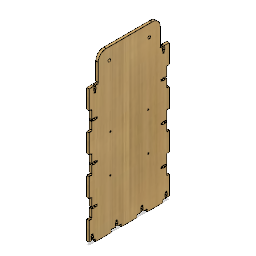
Square-plate-IIIS-electronics-rev1_8mm v1 (Autodesk Fusion 360 design; units mm, degrees)
Autodesk Fusion 360 part; units mm, degrees
sketch "Basic shape" plane through (0, 0, 0) normal (1, 0, 0) x (0, 0, -1)
  line L0 (-117.75, 0) -> (117.75, 0)
  line L1 (117.75, 0) -> (117.75, 417)
  line L2 (117.75, 417) -> (-117.75, 417)
  line L3 (-117.75, 417) -> (-117.75, 0)
  line L4 (-97.5, 417) -> (97.5, 417)
  line L5 (97.5, 417) -> (97.5, 500)
  line L6 (97.5, 500) -> (-97.5, 500)
  line L7 (-97.5, 500) -> (-97.5, 417)
  line L8 (117.75, 0) -> (125.75, 0)
  line L9 (125.75, 0) -> (125.75, 60)
  line L10 (125.75, 60) -> (117.75, 60)
  line L11 (117.75, 60) -> (117.75, 0)
  line L12 (117.75, 119) -> (125.75, 119)
  line L13 (125.75, 119) -> (125.75, 179)
  line L14 (125.75, 179) -> (117.75, 179)
  line L15 (117.75, 179) -> (117.75, 119)
  line L16 (117.75, 238) -> (125.75, 238)
  line L17 (125.75, 238) -> (125.75, 298)
  line L18 (125.75, 298) -> (117.75, 298)
  line L19 (117.75, 298) -> (117.75, 238)
  line L20 (117.75, 357) -> (125.75, 357)
  line L21 (125.75, 357) -> (125.75, 417)
  line L22 (125.75, 417) -> (117.75, 417)
  line L23 (117.75, 417) -> (117.75, 357)
  line L24 (-117.75, 0) -> (-55.75, 0)
  line L25 (-55.75, 0) -> (-55.75, -8)
  line L26 (-55.75, -8) -> (-105.75, -8)
  line L27 (-25, 0) -> (25, 0)
  line L28 (25, 0) -> (25, -8)
  line L29 (25, -8) -> (-25, -8)
  line L30 (-25, -8) -> (-25, 0)
  line L31 (117.75, 0) -> (55.75, 0)
  line L32 (55.75, 0) -> (55.75, -8)
  line L33 (55.75, -8) -> (105.75, -8)
  line L34 (-55.75, -8) -> (-25, -8) construction
  line L35 (25, -8) -> (55.75, -8) construction
  line L36 (-117.75, 0) -> (-125.75, 0)
  line L37 (-125.75, 0) -> (-125.75, 60)
  line L38 (-125.75, 60) -> (-117.75, 60)
  line L39 (-117.75, 60) -> (-117.75, 0)
  line L40 (-117.75, 119) -> (-125.75, 119)
  line L41 (-125.75, 119) -> (-125.75, 179)
  line L42 (-125.75, 179) -> (-117.75, 179)
  line L43 (-117.75, 179) -> (-117.75, 119)
  line L44 (-117.75, 238) -> (-125.75, 238)
  line L45 (-125.75, 238) -> (-125.75, 298)
  line L46 (-125.75, 298) -> (-117.75, 298)
  line L47 (-117.75, 298) -> (-117.75, 238)
  line L48 (-117.75, 357) -> (-125.75, 357)
  line L49 (-125.75, 357) -> (-125.75, 417)
  line L50 (-125.75, 417) -> (-117.75, 417)
  line L51 (-117.75, 417) -> (-117.75, 357)
  line L52 (125.75, 60) -> (125.75, 119) construction
  line L53 (125.75, 179) -> (125.75, 238) construction
  line L54 (-125.75, 60) -> (-125.75, 119) construction
  line L55 (-125.75, 179) -> (-125.75, 238) construction
  line L56 (-105.75, 0) -> (-105.75, -8)
  line L57 (105.75, -8) -> (105.75, 0)
  line L58 (97.5, 417) -> (125.75, 417)
  line L59 (-125.75, 417) -> (-97.5, 417)
  line L60 (-125.75, 357) -> (-125.75, 298) construction
  line L61 (125.75, 357) -> (125.75, 298) construction
  dimension "d1" = 235.5
  dimension "d2" = 417
  dimension "d3" = 83
  dimension "d4" = 195
  dimension "d9" = 60
  dimension "d10" = 60
  dimension "d11" = 60
  dimension "d12" = 60
  dimension "d16" = 50
  dimension "d20" = 8
  dimension "d21" = 8
  dimension "d22" = 60
  dimension "d24" = 60
  dimension "d26" = 60
  dimension "d28" = 60
  dimension "d29" = 8
  dimension "d30" = 8
  dimension "d81" = 8
  dimension "d82" = 20
  dimension "d83" = 20
  dimension "d357" = 50
  dimension "d358" = 50
  dimension "d359" = 30.75
  dimension "d360" = 30.75
  measures "d2" distance of origin
  measures "d22" distance of origin
  measures "d81" distance of L0 L26
  measures "d83" distance of origin
extrude "Extrude1" add sketch "Basic shape" along normal blind 8
sketch "T slots horizontal" plane through (8, 0, 0) normal (1, 0, 0) x (0, 0, -1)
  line L0 (-117.75, 357) -> (-117.75, 298)
  line L1 (-117.75, 298) -> (-125.75, 298)
  line L2 (-125.75, 298) -> (-125.75, 238)
  line L3 (-125.75, 238) -> (-117.75, 238)
  line L4 (-117.75, 238) -> (-117.75, 179)
  line L5 (-117.75, 179) -> (-125.75, 179)
  line L6 (-125.75, 179) -> (-125.75, 119)
  line L7 (-125.75, 119) -> (-117.75, 119)
  line L8 (-117.75, 119) -> (-117.75, 60)
  line L9 (-117.75, 60) -> (-125.75, 60)
  line L10 (-125.75, 60) -> (-125.75, 0)
  line L11 (-125.75, 0) -> (-117.75, 0)
  line L12 (-105.75, -8) -> (-55.75, -8)
  line L13 (-55.75, -8) -> (-55.75, 0)
  line L14 (-117.75, 0) -> (-105.75, 0)
  line L15 (-25, 0) -> (-25, -8)
  line L16 (-25, -8) -> (25, -8)
  line L17 (25, -8) -> (25, 0)
  line L18 (25, 0) -> (55.75, 0)
  line L19 (55.75, 0) -> (55.75, -8)
  line L20 (55.75, -8) -> (105.75, -8)
  line L21 (105.75, 0) -> (125.75, 0)
  line L22 (125.75, 0) -> (125.75, 60)
  line L23 (125.75, 60) -> (117.75, 60)
  line L24 (117.75, 60) -> (117.75, 119)
  line L25 (117.75, 119) -> (125.75, 119)
  line L26 (125.75, 119) -> (125.75, 179)
  line L27 (125.75, 179) -> (117.75, 179)
  line L28 (117.75, 179) -> (117.75, 238)
  line L29 (117.75, 238) -> (125.75, 238)
  line L30 (125.75, 238) -> (125.75, 298)
  line L31 (125.75, 298) -> (117.75, 298)
  line L32 (117.75, 298) -> (117.75, 357)
  line L33 (117.75, 357) -> (125.75, 357)
  line L34 (125.75, 357) -> (125.75, 417)
  line L35 (125.75, 417) -> (97.5, 417)
  line L36 (97.5, 417) -> (97.5, 500)
  line L37 (97.5, 500) -> (-97.5, 500)
  line L38 (-97.5, 500) -> (-97.5, 417)
  line L39 (-97.5, 417) -> (-125.75, 417)
  line L40 (-125.75, 417) -> (-125.75, 357)
  line L41 (-125.75, 357) -> (-117.75, 357)
  line L42 (-41.885, 0) -> (-37.865, 0)
  line L43 (-37.865, 0) -> (-37.865, 17.5)
  line L44 (-37.865, 17.5) -> (-41.885, 17.5)
  line L45 (-41.885, 17.5) -> (-41.885, 0)
  line L46 (-43.355, 12.5) -> (-36.355, 12.5)
  line L47 (-36.355, 12.5) -> (-36.355, 5)
  line L48 (-36.355, 5) -> (-43.355, 5)
  line L49 (-43.355, 5) -> (-43.355, 12.5)
  line L50 (-109.635, 417) -> (-105.615, 417)
  line L51 (-105.615, 417) -> (-105.615, 397)
  line L52 (-105.615, 397) -> (-109.635, 397)
  line L53 (-109.635, 397) -> (-109.635, 417)
  line L54 (-111.105, 412) -> (-104.105, 412)
  line L55 (-104.105, 412) -> (-104.105, 404.5)
  line L56 (-104.105, 404.5) -> (-111.105, 404.5)
  line L57 (-111.105, 404.5) -> (-111.105, 412)
  line L58 (-113.74, 0) -> (-113.74, 17.5)
  line L59 (-117.76, 17.5) -> (-117.76, 0)
  line L60 (-113.74, 17.5) -> (-117.76, 17.5)
  line L61 (-119.23, 5) -> (-119.23, 12.5)
  line L62 (-112.23, 5) -> (-119.23, 5)
  line L63 (-117.76, 0) -> (-113.74, 0)
  line L64 (-112.23, 12.5) -> (-112.23, 5)
  line L65 (-119.23, 12.5) -> (-112.23, 12.5)
  line L66 (-105.75, 0) -> (-105.75, -8)
  line L67 (105.75, -8) -> (105.75, 0)
  line L68 (-55.75, 0) -> (-25, 0)
  dimension "d31" = 4.02
  dimension "d32" = 7
  dimension "d33" = 1.51
  dimension "d34" = 5
  dimension "d35" = 17.5
  dimension "d36" = 7.5
  dimension "d37" = 4.02
  dimension "d38" = 20
  dimension "d39" = 7.5
  dimension "d40" = 1.51
  dimension "d41" = 7
  dimension "d42" = 5
  dimension "d66" = 4.02
  dimension "d67" = 7
  dimension "d68" = 1.51
  dimension "d69" = 5
  dimension "d70" = 17.5
  dimension "d71" = 7.5
  dimension "d80" = 10.125
  dimension "d86" = 14.625
  dimension "d90" = 10
  measures "d33" distance of L43
  measures "d34" distance of origin
  measures "d35" distance of origin
  measures "d68" distance of L58
  measures "d69" distance of origin
  measures "d70" distance of origin
  measures "d90" distance of origin L66
extrude "Extrude2" cut sketch "T slots horizontal" against normal through all contours L39 L50 L51 L53 L54 | L51 L53 L54 L56 | L53 L54 L56 L57 | L51 L54 L55 L56 | L51 L52 L53 L56 | L11 L14 L58 L59 L62 L63 | L59 L61 L62 L65 | L58 L59 L62 L65 | L58 L59 L60 L65 | L58 L62 L64 L65 | L42 L43 L45 L48 L68 | L45 L46 L48 L49 | L43 L45 L46 L48 | L43 L46 L47 L48 | L43 L44 L45 L46
mirror "Mirror1" about plane through (0, 0, 0) normal (0, 0, 1) of "Extrude2"
sketch "T slots vertical" plane through (8, 0, 0) normal (1, 0, 0) x (0, 0, -1)
  line L0 (37.865, 0) -> (37.865, 5)
  line L1 (37.865, 5) -> (36.355, 5)
  line L2 (36.355, 5) -> (36.355, 12.5)
  line L3 (36.355, 12.5) -> (37.865, 12.5)
  line L4 (37.865, 12.5) -> (37.865, 17.5)
  line L5 (37.865, 17.5) -> (41.885, 17.5)
  line L6 (41.885, 17.5) -> (41.885, 12.5)
  line L7 (41.885, 12.5) -> (43.355, 12.5)
  line L8 (43.355, 12.5) -> (43.355, 5)
  line L9 (43.355, 5) -> (41.885, 5)
  line L10 (41.885, 5) -> (41.885, 0)
  line L11 (41.885, 0) -> (55.75, 0)
  line L12 (55.75, 0) -> (55.75, -8)
  line L13 (55.75, -8) -> (105.75, -8)
  line L14 (105.75, 0) -> (113.74, 0)
  line L15 (125.75, 0) -> (125.75, 60)
  line L16 (125.75, 60) -> (117.75, 60)
  line L17 (117.75, 60) -> (117.75, 119)
  line L18 (117.75, 119) -> (125.75, 119)
  line L19 (125.75, 119) -> (125.75, 179)
  line L20 (125.75, 179) -> (117.75, 179)
  line L21 (117.75, 179) -> (117.75, 238)
  line L22 (117.75, 238) -> (125.75, 238)
  line L23 (125.75, 238) -> (125.75, 298)
  line L24 (125.75, 298) -> (117.75, 298)
  line L25 (117.75, 298) -> (117.75, 357)
  line L26 (117.75, 357) -> (125.75, 357)
  line L27 (125.75, 357) -> (125.75, 417)
  line L28 (125.75, 417) -> (109.635, 417)
  line L29 (109.635, 417) -> (109.635, 412)
  line L30 (109.635, 412) -> (111.105, 412)
  line L31 (111.105, 412) -> (111.105, 404.5)
  line L32 (111.105, 404.5) -> (109.635, 404.5)
  line L33 (109.635, 404.5) -> (109.635, 397)
  line L34 (109.635, 397) -> (105.615, 397)
  line L35 (105.615, 397) -> (105.615, 404.5)
  line L36 (105.615, 404.5) -> (104.105, 404.5)
  line L37 (104.105, 404.5) -> (104.105, 412)
  line L38 (104.105, 412) -> (105.615, 412)
  line L39 (105.615, 412) -> (105.615, 417)
  line L40 (105.615, 417) -> (97.5, 417)
  line L41 (97.5, 417) -> (97.5, 500)
  line L42 (97.5, 500) -> (-97.5, 500)
  line L43 (-97.5, 500) -> (-97.5, 417)
  line L44 (-97.5, 417) -> (-105.615, 417)
  line L45 (-105.615, 417) -> (-105.615, 412)
  line L46 (-105.615, 412) -> (-104.105, 412)
  line L47 (-104.105, 412) -> (-104.105, 404.5)
  line L48 (-104.105, 404.5) -> (-105.615, 404.5)
  line L49 (-105.615, 404.5) -> (-105.615, 397)
  line L50 (-105.615, 397) -> (-109.635, 397)
  line L51 (-109.635, 397) -> (-109.635, 404.5)
  line L52 (-109.635, 404.5) -> (-111.105, 404.5)
  line L53 (-111.105, 404.5) -> (-111.105, 412)
  line L54 (-111.105, 412) -> (-109.635, 412)
  line L55 (-109.635, 412) -> (-109.635, 417)
  line L56 (-109.635, 417) -> (-125.75, 417)
  line L57 (-125.75, 417) -> (-125.75, 357)
  line L58 (-125.75, 357) -> (-117.75, 357)
  line L59 (-117.75, 357) -> (-117.75, 298)
  line L60 (-117.75, 298) -> (-125.75, 298)
  line L61 (-125.75, 298) -> (-125.75, 238)
  line L62 (-125.75, 238) -> (-117.75, 238)
  line L63 (-117.75, 238) -> (-117.75, 179)
  line L64 (-117.75, 179) -> (-125.75, 179)
  line L65 (-125.75, 179) -> (-125.75, 119)
  line L66 (-125.75, 119) -> (-117.75, 119)
  line L67 (-117.75, 119) -> (-117.75, 60)
  line L68 (-117.75, 60) -> (-125.75, 60)
  line L69 (-125.75, 60) -> (-125.75, 0)
  line L70 (-125.75, 0) -> (-117.76, 0)
  line L71 (-105.75, -8) -> (-55.75, -8)
  line L72 (-55.75, -8) -> (-55.75, 0)
  line L73 (-55.75, 0) -> (-41.885, 0)
  line L74 (-41.885, 0) -> (-41.885, 5)
  line L75 (-41.885, 5) -> (-43.355, 5)
  line L76 (-43.355, 5) -> (-43.355, 12.5)
  line L77 (-43.355, 12.5) -> (-41.885, 12.5)
  line L78 (-41.885, 12.5) -> (-41.885, 17.5)
  line L79 (-41.885, 17.5) -> (-37.865, 17.5)
  line L80 (-37.865, 17.5) -> (-37.865, 12.5)
  line L81 (-37.865, 12.5) -> (-36.355, 12.5)
  line L82 (-36.355, 12.5) -> (-36.355, 5)
  line L83 (-36.355, 5) -> (-37.865, 5)
  line L84 (-37.865, 5) -> (-37.865, 0)
  line L85 (-37.865, 0) -> (-25, 0)
  line L86 (-25, 0) -> (-25, -8)
  line L87 (-25, -8) -> (25, -8)
  line L88 (25, -8) -> (25, 0)
  line L89 (25, 0) -> (37.865, 0)
  line L90 (-117.75, 91.505) -> (-100.25, 91.505)
  line L91 (-100.25, 91.505) -> (-100.25, 87.495)
  line L92 (-100.25, 87.495) -> (-117.75, 87.495)
  line L93 (-117.75, 87.495) -> (-117.75, 91.505)
  line L94 (-112.75, 93.015) -> (-105.25, 93.015)
  line L95 (-105.25, 93.015) -> (-105.25, 86.015)
  line L96 (-105.25, 86.015) -> (-112.75, 86.015)
  line L97 (-112.75, 86.015) -> (-112.75, 93.015)
  line L98 (113.74, 0) -> (113.74, 5)
  line L99 (113.74, 5) -> (112.23, 5)
  line L100 (112.23, 5) -> (112.23, 12.5)
  line L101 (112.23, 12.5) -> (113.74, 12.5)
  line L102 (113.74, 12.5) -> (113.74, 17.5)
  line L103 (113.74, 17.5) -> (117.76, 17.5)
  line L104 (117.76, 17.5) -> (117.76, 12.5)
  line L105 (117.76, 12.5) -> (119.23, 12.5)
  line L106 (119.23, 12.5) -> (119.23, 5)
  line L107 (119.23, 5) -> (117.76, 5)
  line L108 (117.76, 5) -> (117.76, 0)
  line L109 (117.76, 0) -> (125.75, 0)
  line L110 (-117.76, 0) -> (-117.76, 5)
  line L111 (-117.76, 5) -> (-119.23, 5)
  line L112 (-119.23, 5) -> (-119.23, 12.5)
  line L113 (-119.23, 12.5) -> (-117.76, 12.5)
  line L114 (-117.76, 12.5) -> (-117.76, 17.5)
  line L115 (-117.76, 17.5) -> (-113.74, 17.5)
  line L116 (-113.74, 17.5) -> (-113.74, 12.5)
  line L117 (-113.74, 12.5) -> (-112.23, 12.5)
  line L118 (-112.23, 12.5) -> (-112.23, 5)
  line L119 (-112.23, 5) -> (-113.74, 5)
  line L120 (-113.74, 5) -> (-113.74, 0)
  line L121 (105.75, -8) -> (105.75, 0)
  line L122 (-105.75, 0) -> (-105.75, -8)
  line L123 (-113.74, 0) -> (-105.75, 0)
  dimension "d45" = 1.51
  dimension "d46" = 4.01
  dimension "d47" = 7
  dimension "d48" = 7.5
  dimension "d49" = 5
  dimension "d50" = 17.5
extrude "Extrude3" cut sketch "T slots vertical" against normal through all contours L67 L90 L92 L93 L97 | L90 L92 L95 L97 | L92 L95 L96 L97 | L90 L94 L95 L97 | L90 L91 L92 L95
pattern_linear "R-Pattern1" count 3 spacing 118.6667 along (0, 1, 0) of "Extrude3"
mirror "Mirror2" about plane through (0, 0, 0) normal (0, 0, 1) of "Extrude3", "R-Pattern1"
fillet "Fillet1" radius 25 2 edges at (4, 500, -97.5) (4, 500, 97.5)
sketch "Bar holder" plane through (8, 0, 0) normal (1, 0, 0) x (0, 0, -1)
  arc A0 (-72.5, 500) -> (-97.5, 475) centre (-72.5, 475) ccw
  line L0 (-97.5, 475) -> (-97.5, 417)
  line L1 (-97.5, 417) -> (-105.615, 417)
  line L2 (-105.615, 417) -> (-105.615, 412)
  line L3 (-105.615, 412) -> (-104.105, 412)
  line L4 (-104.105, 412) -> (-104.105, 404.5)
  line L5 (-104.105, 404.5) -> (-105.615, 404.5)
  line L6 (-105.615, 404.5) -> (-105.615, 397)
  line L7 (-105.615, 397) -> (-109.635, 397)
  line L8 (-109.635, 397) -> (-109.635, 404.5)
  line L9 (-109.635, 404.5) -> (-111.105, 404.5)
  line L10 (-111.105, 404.5) -> (-111.105, 412)
  line L11 (-111.105, 412) -> (-109.635, 412)
  line L12 (-109.635, 412) -> (-109.635, 417)
  line L13 (-109.635, 417) -> (-125.75, 417)
  line L14 (-125.75, 417) -> (-125.75, 357)
  line L15 (-125.75, 357) -> (-117.75, 357)
  line L16 (-117.75, 357) -> (-117.75, 328.8383)
  line L17 (-117.75, 328.8383) -> (-112.75, 328.8383)
  line L18 (-112.75, 328.8383) -> (-112.75, 330.3483)
  line L19 (-112.75, 330.3483) -> (-105.25, 330.3483)
  line L20 (-105.25, 330.3483) -> (-105.25, 328.8383)
  line L21 (-105.25, 328.8383) -> (-100.25, 328.8383)
  line L22 (-100.25, 328.8383) -> (-100.25, 324.8283)
  line L23 (-100.25, 324.8283) -> (-105.25, 324.8283)
  line L24 (-105.25, 324.8283) -> (-105.25, 323.3483)
  line L25 (-105.25, 323.3483) -> (-112.75, 323.3483)
  line L26 (-112.75, 323.3483) -> (-112.75, 324.8283)
  line L27 (-112.75, 324.8283) -> (-117.75, 324.8283)
  line L28 (-117.75, 324.8283) -> (-117.75, 298)
  line L29 (-117.75, 298) -> (-125.75, 298)
  line L30 (-125.75, 298) -> (-125.75, 238)
  line L31 (-125.75, 238) -> (-117.75, 238)
  line L32 (-117.75, 238) -> (-117.75, 210.1717)
  line L33 (-117.75, 210.1717) -> (-112.75, 210.1717)
  line L34 (-112.75, 210.1717) -> (-112.75, 211.6817)
  line L35 (-112.75, 211.6817) -> (-105.25, 211.6817)
  line L36 (-105.25, 211.6817) -> (-105.25, 210.1717)
  line L37 (-105.25, 210.1717) -> (-100.25, 210.1717)
  line L38 (-100.25, 210.1717) -> (-100.25, 206.1617)
  line L39 (-100.25, 206.1617) -> (-105.25, 206.1617)
  line L40 (-105.25, 206.1617) -> (-105.25, 204.6817)
  line L41 (-105.25, 204.6817) -> (-112.75, 204.6817)
  line L42 (-112.75, 204.6817) -> (-112.75, 206.1617)
  line L43 (-112.75, 206.1617) -> (-117.75, 206.1617)
  line L44 (-117.75, 206.1617) -> (-117.75, 179)
  line L45 (-117.75, 179) -> (-125.75, 179)
  line L46 (-125.75, 179) -> (-125.75, 119)
  line L47 (-125.75, 119) -> (-117.75, 119)
  line L48 (-117.75, 119) -> (-117.75, 91.505)
  line L49 (-117.75, 91.505) -> (-112.75, 91.505)
  line L50 (-112.75, 91.505) -> (-112.75, 93.015)
  line L51 (-112.75, 93.015) -> (-105.25, 93.015)
  line L52 (-105.25, 93.015) -> (-105.25, 91.505)
  line L53 (-105.25, 91.505) -> (-100.25, 91.505)
  line L54 (-100.25, 91.505) -> (-100.25, 87.495)
  line L55 (-100.25, 87.495) -> (-105.25, 87.495)
  line L56 (-105.25, 87.495) -> (-105.25, 86.015)
  line L57 (-105.25, 86.015) -> (-112.75, 86.015)
  line L58 (-112.75, 86.015) -> (-112.75, 87.495)
  line L59 (-112.75, 87.495) -> (-117.75, 87.495)
  line L60 (-117.75, 87.495) -> (-117.75, 60)
  line L61 (-117.75, 60) -> (-125.75, 60)
  line L62 (-125.75, 60) -> (-125.75, 0)
  line L63 (-125.75, 0) -> (-117.76, 0)
  line L64 (-105.75, -8) -> (-55.75, -8)
  line L65 (-55.75, -8) -> (-55.75, 0)
  line L66 (-55.75, 0) -> (-41.885, 0)
  line L67 (-41.885, 0) -> (-41.885, 5)
  line L68 (-41.885, 5) -> (-43.355, 5)
  line L69 (-43.355, 5) -> (-43.355, 12.5)
  line L70 (-43.355, 12.5) -> (-41.885, 12.5)
  line L71 (-41.885, 12.5) -> (-41.885, 17.5)
  line L72 (-41.885, 17.5) -> (-37.865, 17.5)
  line L73 (-37.865, 17.5) -> (-37.865, 12.5)
  line L74 (-37.865, 12.5) -> (-36.355, 12.5)
  line L75 (-36.355, 12.5) -> (-36.355, 5)
  line L76 (-36.355, 5) -> (-37.865, 5)
  line L77 (-37.865, 5) -> (-37.865, 0)
  line L78 (-37.865, 0) -> (-25, 0)
  line L79 (-25, 0) -> (-25, -8)
  line L80 (-25, -8) -> (25, -8)
  line L81 (25, -8) -> (25, 0)
  line L82 (25, 0) -> (37.865, 0)
  line L83 (37.865, 0) -> (37.865, 5)
  line L84 (37.865, 5) -> (36.355, 5)
  line L85 (36.355, 5) -> (36.355, 12.5)
  line L86 (36.355, 12.5) -> (37.865, 12.5)
  line L87 (37.865, 12.5) -> (37.865, 17.5)
  line L88 (37.865, 17.5) -> (41.885, 17.5)
  line L89 (41.885, 17.5) -> (41.885, 12.5)
  line L90 (41.885, 12.5) -> (43.355, 12.5)
  line L91 (43.355, 12.5) -> (43.355, 5)
  line L92 (43.355, 5) -> (41.885, 5)
  line L93 (41.885, 5) -> (41.885, 0)
  line L94 (41.885, 0) -> (55.75, 0)
  line L95 (55.75, 0) -> (55.75, -8)
  line L96 (55.75, -8) -> (105.75, -8)
  line L97 (105.75, 0) -> (113.74, 0)
  line L98 (125.75, 0) -> (125.75, 60)
  line L99 (125.75, 60) -> (117.75, 60)
  line L100 (117.75, 60) -> (117.75, 87.495)
  line L101 (117.75, 119) -> (125.75, 119)
  line L102 (125.75, 119) -> (125.75, 179)
  line L103 (125.75, 179) -> (117.75, 179)
  line L104 (117.75, 179) -> (117.75, 206.1617)
  line L105 (117.75, 206.1617) -> (112.75, 206.1617)
  line L106 (112.75, 206.1617) -> (112.75, 204.6817)
  line L107 (112.75, 204.6817) -> (105.25, 204.6817)
  line L108 (105.25, 204.6817) -> (105.25, 206.1617)
  line L109 (105.25, 206.1617) -> (100.25, 206.1617)
  line L110 (100.25, 206.1617) -> (100.25, 210.1717)
  line L111 (100.25, 210.1717) -> (105.25, 210.1717)
  line L112 (105.25, 210.1717) -> (105.25, 211.6817)
  line L113 (105.25, 211.6817) -> (112.75, 211.6817)
  line L114 (112.75, 211.6817) -> (112.75, 210.1717)
  line L115 (112.75, 210.1717) -> (117.75, 210.1717)
  line L116 (117.75, 210.1717) -> (117.75, 238)
  line L117 (117.75, 238) -> (125.75, 238)
  line L118 (125.75, 238) -> (125.75, 298)
  line L119 (125.75, 298) -> (117.75, 298)
  line L120 (117.75, 298) -> (117.75, 324.8283)
  line L121 (117.75, 324.8283) -> (112.75, 324.8283)
  line L122 (112.75, 324.8283) -> (112.75, 323.3483)
  line L123 (112.75, 323.3483) -> (105.25, 323.3483)
  line L124 (105.25, 323.3483) -> (105.25, 324.8283)
  line L125 (105.25, 324.8283) -> (100.25, 324.8283)
  line L126 (100.25, 324.8283) -> (100.25, 328.8383)
  line L127 (100.25, 328.8383) -> (105.25, 328.8383)
  line L128 (105.25, 328.8383) -> (105.25, 330.3483)
  line L129 (105.25, 330.3483) -> (112.75, 330.3483)
  line L130 (112.75, 330.3483) -> (112.75, 328.8383)
  line L131 (112.75, 328.8383) -> (117.75, 328.8383)
  line L132 (117.75, 328.8383) -> (117.75, 357)
  line L133 (117.75, 357) -> (125.75, 357)
  line L134 (125.75, 357) -> (125.75, 417)
  line L135 (125.75, 417) -> (109.635, 417)
  line L136 (109.635, 417) -> (109.635, 412)
  line L137 (109.635, 412) -> (111.105, 412)
  line L138 (111.105, 412) -> (111.105, 404.5)
  line L139 (111.105, 404.5) -> (109.635, 404.5)
  line L140 (109.635, 404.5) -> (109.635, 397)
  line L141 (109.635, 397) -> (105.615, 397)
  line L142 (105.615, 397) -> (105.615, 404.5)
  line L143 (105.615, 404.5) -> (104.105, 404.5)
  line L144 (104.105, 404.5) -> (104.105, 412)
  line L145 (104.105, 412) -> (105.615, 412)
  line L146 (105.615, 412) -> (105.615, 417)
  line L147 (105.615, 417) -> (97.5, 417)
  line L148 (97.5, 417) -> (97.5, 475)
  arc A1 (97.5, 475) -> (72.5, 500) centre (72.5, 475) ccw
  line L149 (72.5, 500) -> (-72.5, 500)
  line L150 (-62.5, 462.5) -> (62.5, 462.5) construction
  circle A2 centre (-62.5, 462.5) radius 4
  circle A3 centre (62.5, 462.5) radius 4
  line L151 (0, 500) -> (0, 417) construction
  line L152 (-97.5, 417) -> (97.5, 417) construction
  line L153 (-97.5, 427) -> (97.5, 427) construction
  line L154 (-117.76, 0) -> (-117.76, 5)
  line L155 (-117.76, 5) -> (-119.23, 5)
  line L156 (-119.23, 5) -> (-119.23, 12.5)
  line L157 (-119.23, 12.5) -> (-117.76, 12.5)
  line L158 (-117.76, 12.5) -> (-117.76, 17.5)
  line L159 (-117.76, 17.5) -> (-113.74, 17.5)
  line L160 (-113.74, 17.5) -> (-113.74, 12.5)
  line L161 (-113.74, 12.5) -> (-112.23, 12.5)
  line L162 (-112.23, 12.5) -> (-112.23, 5)
  line L163 (-112.23, 5) -> (-113.74, 5)
  line L164 (-113.74, 5) -> (-113.74, 0)
  line L165 (113.74, 0) -> (113.74, 5)
  line L166 (113.74, 5) -> (112.23, 5)
  line L167 (112.23, 5) -> (112.23, 12.5)
  line L168 (112.23, 12.5) -> (113.74, 12.5)
  line L169 (113.74, 12.5) -> (113.74, 17.5)
  line L170 (113.74, 17.5) -> (117.76, 17.5)
  line L171 (117.76, 17.5) -> (117.76, 12.5)
  line L172 (117.76, 12.5) -> (119.23, 12.5)
  line L173 (119.23, 12.5) -> (119.23, 5)
  line L174 (119.23, 5) -> (117.76, 5)
  line L175 (117.76, 5) -> (117.76, 0)
  line L176 (117.76, 0) -> (125.75, 0)
  line L177 (-105.75, 0) -> (-105.75, -8)
  line L178 (105.75, -8) -> (105.75, 0)
  line L179 (117.75, 87.495) -> (112.75, 87.495)
  line L180 (112.75, 87.495) -> (112.75, 86.015)
  line L181 (112.75, 86.015) -> (105.25, 86.015)
  line L182 (105.25, 86.015) -> (105.25, 87.495)
  line L183 (105.25, 87.495) -> (100.25, 87.495)
  line L184 (100.25, 87.495) -> (100.25, 91.505)
  line L185 (100.25, 91.505) -> (105.25, 91.505)
  line L186 (105.25, 91.505) -> (105.25, 93.015)
  line L187 (105.25, 93.015) -> (112.75, 93.015)
  line L188 (112.75, 93.015) -> (112.75, 91.505)
  line L189 (112.75, 91.505) -> (117.75, 91.505)
  line L190 (117.75, 91.505) -> (117.75, 119)
  line L191 (-113.74, 0) -> (-105.75, 0)
  dimension "d58" = 125
  dimension "d59" = 8
  dimension "d60" = 8
  dimension "d62" = 10
  dimension "d63" = 75
  dimension "d64" = 37.5
  measures "d59" diameter of A2
  measures "d60" diameter of A3
  measures "d62" distance of L152 L153
  measures "d63" distance of L149 L153
  measures "d64" distance of L149
extrude "Extrude4" cut sketch "Bar holder" against normal through all contours A2 | A3
sketch "Electronics" plane through (8, 0, 0) normal (1, 0, 0) x (0, 0, -1)
  line L0 (-59.5, 268) -> (59.5, 268) construction
  line L1 (59.5, 268) -> (59.5, 149) construction
  line L2 (59.5, 149) -> (-59.5, 149) construction
  line L3 (-59.5, 149) -> (-59.5, 268) construction
  circle A0 centre (-59.5, 268) radius 2
  circle A1 centre (59.5, 268) radius 2
  circle A2 centre (-59.5, 149) radius 2
  circle A3 centre (59.5, 149) radius 2
  dimension "d75" = 4
  dimension "d76" = 4
  dimension "d77" = 4
  dimension "d78" = 4
  dimension "d361" = 119
  dimension "d362" = 119
  dimension "d363" = 149
  measures "d75" diameter of A0
  measures "d76" diameter of A1
  measures "d77" diameter of A3
  measures "d78" diameter of A2
extrude "Extrude5" cut sketch "Electronics" against normal through all
hole "Hole1" at (8, 180.4142, -119.1642) direction (-1, 0, 0) diameter 4 end up to surface (8 mm away)
hole "Hole2" at (8, 355.5858, 119.1642) direction (-1, 0, 0) diameter 4 end up to surface (8 mm away)
hole "Hole3" at (8, 117.5858, 119.1642) direction (-1, 0, 0) diameter 4 end up to surface (8 mm away)
hole "Hole4" at (8, 299.4142, -119.1642) direction (-1, 0, 0) diameter 4 end up to surface (8 mm away)
hole "Hole5" at (8, -1.4142, 54.3358) direction (-1, 0, 0) diameter 4 end up to surface (8 mm away)
hole "Hole6" at (8, 355.5858, -119.1642) direction (-1, 0, 0) diameter 4 end up to surface (8 mm away)
hole "Hole7" at (8, 236.5858, -119.1642) direction (-1, 0, 0) diameter 4 end up to surface (8 mm away)
hole "Hole8" at (8, -1.4142, 26.4142) direction (-1, 0, 0) diameter 4 end up to surface (8 mm away)
hole "Hole9" at (8, -1.4142, -107.1642) direction (-1, 0, 0) diameter 4 end up to surface (8 mm away)
hole "Hole10" at (8, 418.4142, 98.9142) direction (-1, 0, 0) diameter 4 end up to surface (8 mm away)
hole "Hole11" at (8, 61.4142, 119.1642) direction (-1, 0, 0) diameter 4 end up to surface (8 mm away)
hole "Hole12" at (8, 236.5858, 119.1642) direction (-1, 0, 0) diameter 4 end up to surface (8 mm away)
hole "Hole13" at (8, 299.4142, 119.1642) direction (-1, 0, 0) diameter 4 end up to surface (8 mm away)
hole "Hole14" at (8, -1.4142, -54.3358) direction (-1, 0, 0) diameter 4 end up to surface (8 mm away)
hole "Hole15" at (8, -1.4142, -26.4142) direction (-1, 0, 0) diameter 4 end up to surface (8 mm away)
hole "Hole16" at (8, -1.4142, 107.1642) direction (-1, 0, 0) diameter 4 end up to surface (8 mm away)
hole "Hole17" at (8, 61.4142, -119.1642) direction (-1, 0, 0) diameter 4 end up to surface (8 mm away)
hole "Hole18" at (8, 117.5858, -119.1642) direction (-1, 0, 0) diameter 4 end up to surface (8 mm away)
hole "Hole19" at (8, 180.4142, 119.1642) direction (-1, 0, 0) diameter 4 end up to surface (8 mm away)
hole "Hole20" at (8, 418.4142, -98.9142) direction (-1, 0, 0) diameter 4 end up to surface (8 mm away)
equation "pannel_thickness = 8 mm"
equation "d7 = pannel_thickness"
equation "d16 = Square_joint_thickness"
equation "d20 = pannel_thickness"
equation "d21 = pannel_thickness"
equation "d29 = pannel_thickness"
equation "d30 = pannel_thickness"
equation "d31 = tslot_diameter + 0.02 mm"
equation "d33 = ( ( 7 mm - tslot_diameter ) / 2 ) + 0.01 mm"
equation "d37 = tslot_diameter + 0.02 mm"
equation "d40 = ( ( 7 mm - tslot_diameter ) / 2 ) + 0.01 mm"
equation "d45 = ( ( 7 mm - tslot_diameter ) / 2 ) + 0.01 mm"
equation "d46 = tslot_diameter + 0.01 mm"
equation "d64 = ( 75 / 2 ) * 1 mm"
equation "d66 = tslot_diameter + 0.02 mm"
equation "d68 = ( ( 7 mm - tslot_diameter ) / 2 ) + 0.01 mm"
equation "d81 = pannel_thickness"
equation "d82 = pannel_thickness + 12 mm"
equation "d83 = pannel_thickness + 12 mm"
equation "tslot_diameter = 4 mm"
equation "dbToolDia = 4 mm"
equation "dbOffset = 0 mm" comment "Do NOT change formula"
equation "dbRadius = ( dbToolDia + dbOffset ) / 2" comment "Do NOT change formula"
equation "dbMinPercent = 10"
equation "dbHoleOffset = dbRadius / sqrt(2)" comment "Do NOT change formula"
equation "d257 = dbRadius * 2"
equation "d259 = dbHoleOffset"
equation "d260 = dbHoleOffset"
equation "d262 = dbRadius * 2"
equation "d264 = dbHoleOffset"
equation "d265 = dbHoleOffset"
equation "d267 = dbRadius * 2"
equation "d269 = dbHoleOffset"
equation "d270 = dbHoleOffset"
equation "d272 = dbRadius * 2"
equation "d274 = dbHoleOffset"
equation "d275 = dbHoleOffset"
equation "d277 = dbRadius * 2"
equation "d279 = dbHoleOffset"
equation "d280 = dbHoleOffset"
equation "d282 = dbRadius * 2"
equation "d284 = dbHoleOffset"
equation "d285 = dbHoleOffset"
equation "d287 = dbRadius * 2"
equation "d289 = dbHoleOffset"
equation "d290 = dbHoleOffset"
equation "d292 = dbRadius * 2"
equation "d294 = dbHoleOffset"
equation "d295 = dbHoleOffset"
equation "d297 = dbRadius * 2"
equation "d299 = dbHoleOffset"
equation "d300 = dbHoleOffset"
equation "d302 = dbRadius * 2"
equation "d304 = dbHoleOffset"
equation "d305 = dbHoleOffset"
equation "d307 = dbRadius * 2"
equation "d309 = dbHoleOffset"
equation "d310 = dbHoleOffset"
equation "d312 = dbRadius * 2"
equation "d314 = dbHoleOffset"
equation "d315 = dbHoleOffset"
equation "d317 = dbRadius * 2"
equation "d319 = dbHoleOffset"
equation "d320 = dbHoleOffset"
equation "d322 = dbRadius * 2"
equation "d324 = dbHoleOffset"
equation "d325 = dbHoleOffset"
equation "d327 = dbRadius * 2"
equation "d329 = dbHoleOffset"
equation "d330 = dbHoleOffset"
equation "d332 = dbRadius * 2"
equation "d334 = dbHoleOffset"
equation "d335 = dbHoleOffset"
equation "d337 = dbRadius * 2"
equation "d339 = dbHoleOffset"
equation "d340 = dbHoleOffset"
equation "d342 = dbRadius * 2"
equation "d344 = dbHoleOffset"
equation "d345 = dbHoleOffset"
equation "d347 = dbRadius * 2"
equation "d349 = dbHoleOffset"
equation "d350 = dbHoleOffset"
equation "d352 = dbRadius * 2"
equation "d354 = dbHoleOffset"
equation "d355 = dbHoleOffset"
equation "Square_joint_thickness = 50 mm"
